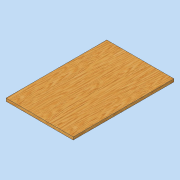
# Autodesk Inventor part: plywood
Saved by Autodesk Inventor 2019 (Build 230136000, 136)
## iProperties
Created: 2019-12-05
Part Number: plywood
Material: Plywood, Finish
Document SubType Name: Modeling
Designer: qitilab4
Density: 0.552 g/cm^3
Appearance: Plywood - New
Author: qitilab4
Autodesk Inventor part; units mm, degrees
ref_plane "YZ Plane" through (0, 0, 0) normal (1, 0, 0) x (0, 1, 0)
ref_plane "XZ Plane" through (0, 0, 0) normal (0, 1, 0) x (-1, 0, 0)
ref_plane "XY Plane" through (0, 0, 0) normal (0, 0, 1) x (1, 0, 0)
sketch "Sketch1" plane through (0, 0, 0) normal (0, 1, 0) x (-1, 0, 0)
  line L0 (-304.8, 457.2) -> (304.8, 457.2)
  line L1 (304.8, 457.2) -> (304.8, -457.2)
  line L2 (304.8, -457.2) -> (-304.8, -457.2)
  line L3 (-304.8, -457.2) -> (-304.8, 457.2)
  line L4 (-304.8, 457.2) -> (304.8, -457.2) construction
  line L5 (304.8, 457.2) -> (-304.8, -457.2) construction
  point P0 (0, 0)
  dimension "d0" = 609.6
  dimension "d1" = 914.4
  constraints: 12 end point, 2 midpoint, 2 parallel, 1 horizontal, 1 perpendicular
  measures "d0" distance of L1.end L2.end
  measures "d1" distance of L0.end L1.end
extrude "Extrusion1" add sketch "Sketch1" along normal blind 25.4
body "Solid1"
